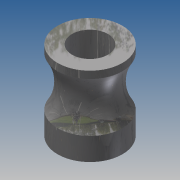
# Autodesk Inventor part: MK8_Drive_gear
Saved by Autodesk Inventor 2015 SP1 (Build 190203100, 203)
## iProperties
Created: 2015-01-28
Part Number: MK8_Drive_gear
Material: Stahl, Kohlenstoff
Document SubType Name: Modeling
Designer: Marc
Mass: 2.87534 g
Surface Area: 5.52653 cm^2
Volume: 0.366285 cm^3
Density: 7.85 g/cm^3
Appearance: Halbpoliert
Author: Marc
Autodesk Inventor part; units mm, degrees
ref_plane "YZ Plane" through (0, 0, 0) normal (1, 0, 0) x (0, 1, 0)
ref_plane "XZ Plane" through (0, 0, 0) normal (0, 1, 0) x (-1, 0, 0)
ref_plane "XY Plane" through (0, 0, 0) normal (0, 0, 1) x (1, 0, 0)
sketch "Skizze1" plane through (0, 0, 0) normal (0, 0, 1) x (1, 0, 0)
  circle A0 centre (0, 0) radius 4.5
  dimension "d0" = 9
  constraints: 1 centre point, 1 coincident
  measures "d0" diameter of A0
extrude "Extrusion1" add sketch "Skizze1" along normal blind 11
sketch "Skizze2" plane through (0, 0, 11) normal (0, 0, 1) x (1, 0, 0)
  circle A0 centre (0, 0) radius 2.5
  dimension "d3" = 5
  constraints: 1 centre point, 1 coincident
  measures "d3" diameter of A0
extrude "Extrusion2" cut sketch "Skizze2" against normal blind 11
sketch "Skizze5" plane through (0, 0, 0) normal (0, 1, 0) x (-1, 0, 0)
  line L0 (4.5, 11) -> (-4.5, 11) projected
  line L1 (-4.5, 0) -> (4.5, 0) projected
  line L2 (4.5, 0) -> (4.5, 11) projected
  line L3 (-4.5, 0) -> (-4.5, 11) projected
  arc A0 (4.5, 10) -> (4.5, 3.1436) centre (10, 6.5718) ccw
  line L4 (4.5, 11) -> (-4.5, 11) projected
  line L5 (3.5, 11) -> (3.5, 0)
  line L6 (-4.5, 0) -> (4.5, 0) projected
  line L7 (4.5, 3.1436) -> (4.5, 10)
  line L8 (0, -2.2) -> (0, 13.2) projected
  point P0 (0, 0)
  dimension "d12" = 1
  dimension "d13" = 5.5
  constraints: 4 end point, 4 point on line, 2 point on circle, 1 centre point, 1 collinear, 1 perpendicular
  measures "d12" distance from line of L0 L7.end
  measures "d13" distance from line of L2 A0.centre
revolve "Umdrehung1" cut sketch "Skizze5" angle 360 about axis through (0, 0, -10) along (0, 0, 1) contours L2 A0
